medal_hanger (Autodesk Fusion 360 design; units mm, degrees)
Autodesk Fusion 360 part; units mm, degrees
sketch "Sketch1" plane through (0, 0, 0) normal (0, 1, 0) x (1, 0, 0)
  line L0 (0, 0) -> (20, 0)
  line L1 (20, 0) -> (20, -30)
  line L2 (20, -30) -> (0, -30)
  line L3 (0, -30) -> (0, 0)
  arc A0 (0, 0) -> (20, 0) centre (10, 0) ccw
  circle A1 centre (10, -22) radius 1.25
  line L4 (10, 0) -> (10, -30) construction
  line L5 (0, -22) -> (20, -22) construction
  dimension "d1" = 20
  dimension "d2" = 30
  dimension "d3" = 2.5
  dimension "d4" = 8
  constraint horizontal L0
  constraint vertical L1
  constraint horizontal L2
  constraint vertical L3
  constraint coincident L0.start L3.end
  constraint tangent L1 A0
  constraint tangent L3 A0
  constraint coincident A0.centre L4.start
  constraint midpoint L2 L4.end
  constraint coincident L3 L5.start
  constraint coincident L1 L5.end
  constraint perpendicular L1 L5
  constraint coincident A1.centre L4
  constraint coincident A1.centre L5
  measures "d1" distance of L1.end L2.end
  measures "d2" distance of L0.end L1.end
  measures "d3" diameter of A1
  measures "d4" distance of L2 L5
extrude "Extrude1" add sketch "Sketch1" against normal blind 4 contours L1 L2 L3 A0
extrude "Extrude2" add sketch "Sketch1" along normal blind 35 and the other way blind 4 contours L0 A0
fillet "Fillet1" radius 7 2 edges at (0, -2, 30) (20, -2, 30)
ref_plane "WorkPlane1" through (10, 39, 5) normal (0, 1, 0) x (1, 0, 0)
sketch "Sketch2" plane through (0, 39, 0) normal (0, 1, 0) x (1, 0, 0)
  arc A0 (0, 0) -> (20, 0) centre (10, 0) ccw
  arc A1 (-3.2515, 0) -> (23.2515, 0) centre (10, 0) ccw
  line L0 (-3.2515, 0) -> (23.2515, 0)
  dimension "d14" = 3.2515
  constraint coincident A0.start origin
  constraint horizontal L0
loft "Loft1" add profiles "Sketch2" section 1 face at (11.7598, 35, 5.4775) section 2
fillet "Fillet2" radius 1.5 2 edges at (10, 35, 10) (10, 39, 13.2515)
